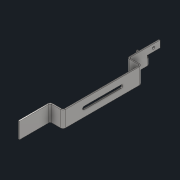
# Autodesk Inventor part: PistaMecBloq2
Saved by Autodesk Inventor 2021 (Build 250183000, 183)
## iProperties
Created: 2021-06-10
Part Number: PistaMecBloq2
Material: Stainless Steel
Document SubType Name: Sheet Metal
Designer: GABRIEL LOL
Density: 8 g/cm^3
Sheet Metal Rule: Por defecto_mm
Appearance: Semi-Polished
Flat Pattern Width: 2.5 cm
Flat Pattern Length: 25.4096 cm
Flat Pattern Area: 63.5239 cm^2
Sheet Metal Width: 25.000 mm
Sheet Metal Length: 254.096 mm
Sheet Metal Area: 6352.389 mm^2
Author: GABRIEL LOL
Autodesk Inventor part; units mm, degrees
ref_plane "YZ Plane" through (0, 0, 0) normal (1, 0, 0) x (0, 1, 0)
ref_plane "XZ Plane" through (0, 0, 0) normal (0, 1, 0) x (-1, 0, 0)
ref_plane "XY Plane" through (0, 0, 0) normal (0, 0, 1) x (1, 0, 0)
sketch "Sketch1" plane through (0, 0, 0) normal (0, 1, 0) x (-1, 0, 0)
  line L0 (0, 0) -> (-200, 0) construction
  line L1 (-200, 0) -> (-150, 0)
  line L2 (-150, 0) -> (-150, -20)
  line L3 (-150, -20) -> (-30, -20)
  line L4 (-30, -20) -> (-30, 0)
  line L5 (-30, 0) -> (0, 0)
  dimension "d0" = 200
  dimension "d1" = 50
  dimension "d2" = 20
  dimension "d3" = 120
  dimension "d4" = 20
  measures "d0" distance of L0.start L0.end
  measures "d1" distance of L0.end L1.end
  measures "d2" distance of L1.end L2.end
  measures "d3" distance of L2.end L3.end
  measures "d4" distance of L3.end L4.end
contour flange "Contour Flange1" sketch "Sketch1" thickness 2 bend radius 2 width 25 along (0, 1, 0) mid plane no both sides no wall seen from (175, 0, 0) lies toward (0, 0, -1) curves L1 L2 L3 L4 L5
bend "Bend1"
corner "Corner1"
sketch "Sketch2" plane through (148, 25, -22) normal (0, 0, -1) x (-1, 0, 0)
  line L0 (116, 0) -> (116, -25) projected
  line L1 (0, 0) -> (116, 0) projected
  line L2 (0, 0) -> (0, -25) projected
  line L3 (0, -25) -> (116, -25) projected
  line L4 (58, -12.5) -> (29, -12.5) construction
  line L5 (0, -25) -> (0, 0) projected
  line L6 (29, -12.5) -> (87, -12.5) construction
  line L7 (87, -12.5) -> (29, -12.5) construction
  line L8 (87, -10) -> (29, -10)
  line L9 (29, -15) -> (87, -15)
  arc A0 (87, -15) -> (87, -10) centre (87, -12.5) ccw
  arc A1 (29, -10) -> (29, -15) centre (29, -12.5) ccw
  point P0 (148, -25)
  point P1 (58, -12.5)
  dimension "d16" = 29
  dimension "d17" = 58
  dimension "d18" = 5
  constraints: 12 end point, 4 point on circle, 4 tangent, 2 centre point, 1 collinear, 1 midpoint, 1 parallel, 1 perpendicular, 1 point on line
  measures "d16" distance of L4.start L4.end
  measures "d17" distance of L4.end L6.end
  measures "d18" diameter of A1
extrude "Extrusion1" cut sketch "Sketch2" against normal blind 10 contours A0 L9 A1 L8
sketch "Sketch4" plane through (0, 0, 0) normal (0, 0, 1) x (1, 0, 0)
  line L0 (0, 0) -> (0, 25) construction
  line L1 (0, 12.5) -> (-20, 12.5) construction
  line L2 (-20, 0) -> (-20, 25) construction
  line L3 (-20, 12.5) -> (-20, 14.5) construction
  line L4 (-20, 12.5) -> (-20, 10.5) construction
  line L5 (0, 0) -> (-20, 0)
  line L6 (-20, 0) -> (-20, 10.5)
  line L7 (-20, 10.5) -> (0, 10.5)
  line L8 (0, 10.5) -> (0, 14.5)
  line L9 (0, 14.5) -> (-20, 14.5)
  line L10 (-20, 14.5) -> (-20, 25)
  line L11 (0, 25) -> (-20, 25)
  line L12 (0, 14.5) -> (0, 25)
  line L13 (0, 0) -> (0, 10.5)
  dimension "d21" = 20
  dimension "d22" = 2
  dimension "d23" = 2
  measures "d21" distance of L1.start L1.end
  measures "d22" distance of L1.end L3.end
  measures "d23" distance of L1.end L4.end
sheet face with bend "Face1" sketch "Sketch4" thickness 2 toward (0, 0, -1) bend radius 2
bend "Bend2"
sketch "Sketch5" plane through (26, 0, 0) normal (0, 0, 1) x (1, 0, 0)
  line L0 (-26, 10.5) -> (-26, 14.5) projected
  line L1 (-26, 10.5) -> (-26, 0)
  constraints: 2 end point, 1 vertical
fold "Fold1" angle 90 bend radius 2 thickness 2 k factor 0.44 line from (0, 10.5, 0) to (0, 0, 0) line at bend end moving side (1, 0, 0) folds toward (0, 0, 1)
sketch "Sketch6" plane through (-2.5239, 14.5, -18) normal (-1, 0, 0) x (0, 0, 1)
  line L0 (20, -14.5) -> (20, -4) projected
  line L1 (46, -14.5) -> (20, -14.5) projected
  line L2 (46, -14.5) -> (46, 10.5) projected
  line L3 (0, 10.5) -> (46, 10.5) projected
  line L4 (0, 10.5) -> (0, 0) projected
  line L5 (0, 0) -> (20, 0) projected
  line L6 (20, -4) -> (20, 0) projected
  circle A0 centre (10, 5.25) radius 2.5
  point P0 (18, -14.5)
  dimension "d35" = 5
  constraints: 1 centre point
  measures "d35" diameter of A0
hole "Hole1" at (-2.5239, 19.75, -8) direction (1, 0, 0) diameter 4 depth 2
equation "\"d5\" = Thickness"
equation "\"d29\" = BendReliefWidth"
equation "\"d31\" = MinimumRemnant"
equation "\"d32\" = TransitionRadius"
equation "\"d34\" = BendRadius"
equation "\"d41\" = Thickness"
equation "\"d6\" = BendReliefWidth"
equation "\"d7\" = BendReliefDepth"
equation "\"d8\" = MinimumRemnant"
equation "\"d9\" = TransitionRadius"
equation "\"d11\" = BendRadius"
equation "\"d13\" = CornerReliefSize"
equation "\"d14\" = GapSize"
equation "\"d15\" = JacobiRadiusSize"
equation "\"d24\" = BendRadius"
equation "\"d25\" = BendReliefWidth"
equation "\"d27\" = MinimumRemnant"
equation "\"d26\" = BendReliefDepth"
equation "\"d28\" = TransitionRadius"
equation "\"BendRadius\" = Thickness"
equation "\"BendReliefWidth\" = Thickness"
equation "\"BendReliefDepth\" = 0.5 * Thickness"
equation "\"CornerReliefSize\" = 4 * Thickness"
equation "\"MinimumRemnant\" = 2 * Thickness"
equation "\"TransitionRadius\" = BendRadius"
equation "\"JacobiRadiusSize\" = BendRadius"
equation "\"GapSize\" = Thickness"
equation "\"Thickness\" = 2"
body "Solid1"
